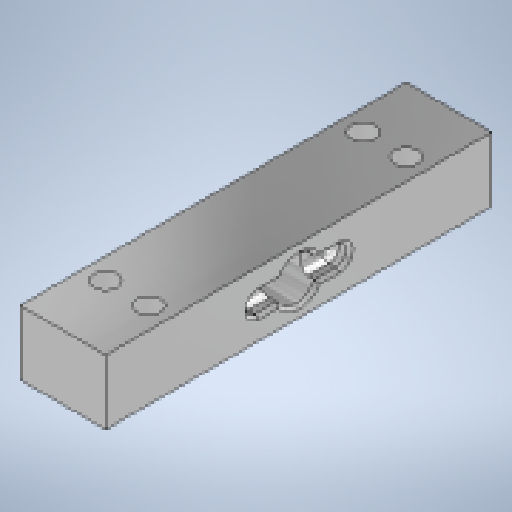
# Autodesk Inventor part: Rack - Top
Saved by Autodesk Inventor 2023.2 (Build 272271000, 271)
## iProperties
Created: 2024-01-12
Part Number: Rack - Top
Material: Aluminum 6061
Document SubType Name: Modeling
Designer: Nathan Cai
Density: 2.7 g/cm^3
Appearance: Aluminum - Flat
Mass: 16.3999 g
Surface Area: 33.3881 cm^2
Volume: 6.07403 cm^3
Author: Nathan Cai
Autodesk Inventor part; units mm, degrees
ref_plane "YZ Plane" through (0, 0, 0) normal (1, 0, 0) x (0, 1, 0)
ref_plane "XZ Plane" through (0, 0, 0) normal (0, 1, 0) x (-1, 0, 0)
ref_plane "XY Plane" through (0, 0, 0) normal (0, 0, 1) x (1, 0, 0)
sketch "Sketch1" plane through (0, 0, 0) normal (0, 1, 0) x (-1, 0, 0)
  line L0 (-3.175, 17.4625) -> (3.175, 17.4625) construction
  line L1 (3.175, 17.4625) -> (3.175, -17.4625) construction
  line L2 (3.175, -17.4625) -> (-3.175, -17.4625) construction
  line L3 (-3.175, -17.4625) -> (-3.175, 17.4625) construction
  line L4 (-3.175, 17.4625) -> (3.175, -17.4625) construction
  line L5 (3.175, 17.4625) -> (-3.175, -17.4625) construction
  circle A0 centre (3.175, 17.4625) radius 1.7526
  circle A1 centre (3.175, -17.4625) radius 1.7526
  circle A2 centre (-3.175, 17.4625) radius 1.7526
  circle A3 centre (-3.175, -17.4625) radius 1.7526
  line L6 (-6.35, 28.575) -> (6.35, 28.575)
  line L7 (6.35, 28.575) -> (6.35, -28.575)
  line L8 (6.35, -28.575) -> (-6.35, -28.575)
  line L9 (-6.35, -28.575) -> (-6.35, 28.575)
  line L10 (-6.35, 28.575) -> (6.35, -28.575) construction
  line L11 (6.35, 28.575) -> (-6.35, -28.575) construction
  point P0 (0, 0)
  dimension "d0" = 6.35
  dimension "d1" = 34.925
  dimension "d2" = 3.5052
  dimension "d5" = 34.925
  dimension "d8" = 6.35
  dimension "d11" = 12.7
  dimension "d12" = 57.15
  constraints: 24 end point, 4 centre point, 4 midpoint, 4 parallel, 3 horizontal, 2 perpendicular, 1 coincident, 1 vertical, 6 other
  measures "d0" distance of L1.end L2.end
  measures "d1" distance of L0.end L1.end
  measures "d2" diameter of A0
  measures "d5" distance of A0.centre A1.centre
  measures "d8" distance of A0.centre A2.centre
  measures "d11" distance of L7.end L8.end
  measures "d12" distance of L6.end L7.end
extrude "Extrusion1" add sketch "Sketch1" along normal blind 9.525
sketch "Sketch2" plane through (6.35, 0, 28.575) normal (1, 0, 0) x (0, 0, -1)
  line L0 (28.575, 0) -> (28.575, 9.525) construction
  line L1 (57.15, 9.525) -> (0, 9.525) projected
  circle A0 centre (28.575, 4.7625) radius 3.175
  line L2 (0, 0) -> (57.15, 0) projected
  point P0 (25.4, 0)
  point P1 (16.2434, 0)
  dimension "d15" = 6.35
  dimension "d16" = 4.7625
  constraints: 2 end point, 2 midpoint, 1 centre point
  measures "d15" diameter of A0
  measures "d16" distance from line of L2 A0.centre
extrude "Extrusion2" cut sketch "Sketch2" against normal through all
sketch "Sketch5" plane through (6.35, 0, 28.575) normal (1, 0, 0) x (0, 0, -1)
  line L0 (0, 0) -> (0, 9.525) projected
  line L1 (0, 4.7625) -> (57.15, 4.7625) construction
  line L2 (57.15, 0) -> (57.15, 9.525) projected
  line L3 (22.575, 4.7625) -> (34.575, 4.7625) construction
  line L4 (22.575, 3.2625) -> (34.575, 3.2625)
  line L5 (34.575, 6.2625) -> (22.575, 6.2625)
  arc A0 (22.575, 6.2625) -> (22.575, 3.2625) centre (22.575, 4.7625) ccw
  arc A1 (34.575, 3.2625) -> (34.575, 6.2625) centre (34.575, 4.7625) ccw
  point P0 (28.575, 0)
  point P1 (28.575, 4.7625)
  dimension "d29" = 3
  dimension "d30" = 12
  constraints: 10 end point, 4 midpoint, 4 point on circle, 4 tangent, 2 centre point, 1 parallel, 1 point on line
  measures "d29" diameter of A1
  measures "d30" distance of L3.start L3.end
extrude "Extrusion5" cut sketch "Sketch5" against normal blind 3
fillet "Fillet3" radius 1.5 6 edges at (3.35, 6.2625, 4.3992) (3.35, 3.2625, 4.3992) (3.35, 4.7625, 7.5) (3.35, 4.7625, -7.5) (3.35, 3.2625, -4.3992) (3.35, 6.2625, -4.3992)
chamfer "Chamfer1" distance 0.5 angle 45 8 edges at (6.35, 3.2625, -4.3992) (6.35, 4.7625, -7.5) (6.35, 6.2625, -4.3992) (6.35, 7.9375, 0) (6.35, 6.2625, 4.3992) (6.35, 4.7625, 7.5) (6.35, 3.2625, 4.3992) (6.35, 1.5875, 0)
equation "\"d5\" = d1"
equation "\"d8\" = d0"
body "Solid1"
